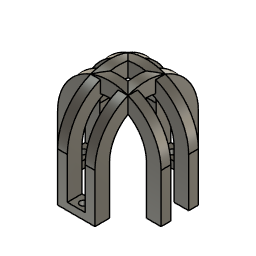
final motor guard (Autodesk Fusion 360 design; units mm, degrees)
Autodesk Fusion 360 part; units mm, degrees
note: some values were not read from the file. Chosen so that the rebuilt part matches the saved one: which bodies a step acts on.
sketch "Sketch1" plane through (0, 0, 0) normal (0, 0, 1) x (1, 0, 0) in component "guard"
  line L0 (-7.5594, 18.25) -> (-18.25, 7.5594)
  line L1 (-18.25, 7.5594) -> (-18.25, -7.5594)
  line L2 (-18.25, -7.5594) -> (-7.5594, -18.25)
  line L3 (-7.5594, -18.25) -> (7.5594, -18.25)
  line L4 (7.5594, -18.25) -> (18.25, -7.5594)
  line L5 (18.25, -7.5594) -> (18.25, 7.5594)
  line L6 (18.25, 7.5594) -> (7.5594, 18.25)
  line L7 (7.5594, 18.25) -> (-7.5594, 18.25)
  circle A0 centre (0, -18.25) radius 1.5
  line L8 (0, 0) -> (0, -18.25)
  circle A1 centre (18.25, 0) radius 1.5
  circle A2 centre (0, 18.25) radius 1.5
  circle A3 centre (-18.25, 0) radius 1.5
  line L9 (0, -18.25) -> (0, -21.25)
  line L10 (0, -21.25) -> (7.663, -21.25)
  line L11 (0, -21.25) -> (-7.663, -21.25)
  line L12 (21.25, 0) -> (21.25, -7.663)
  line L13 (21.25, 0) -> (21.25, 7.663)
  line L14 (18.25, 0) -> (21.25, 0)
  line L15 (0, 21.25) -> (7.663, 21.25)
  line L16 (0, 21.25) -> (-7.663, 21.25)
  line L17 (0, 18.25) -> (0, 21.25)
  line L18 (-21.25, 0) -> (-21.25, 7.663)
  line L19 (-21.25, 0) -> (-21.25, -7.663)
  line L20 (-18.25, 0) -> (-21.25, 0)
  line L21 (7.663, -21.25) -> (7.663, -15.25)
  line L22 (-7.663, -21.25) -> (-7.663, -15.25)
  line L23 (0, -18.25) -> (0, -15.25)
  line L24 (-7.663, -15.25) -> (-3.663, -15.25)
  line L25 (-3.663, -15.25) -> (-3.663, -21.25)
  line L26 (0, -18.25) -> (-3, -18.25)
  line L27 (7.663, -15.25) -> (3.663, -15.25)
  line L28 (3.663, -15.25) -> (3.663, -21.25)
  line L29 (-3.663, -15.25) -> (3.663, -15.25)
  line L30 (21.25, -7.663) -> (15.25, -7.663)
  line L31 (15.25, -7.663) -> (15.25, -3.663)
  line L32 (15.25, -3.663) -> (21.25, -3.663)
  line L33 (21.25, 0) -> (21.25, -7.663)
  line L34 (15.25, 7.663) -> (15.25, 3.663)
  line L35 (21.25, 7.663) -> (15.25, 7.663)
  line L36 (15.25, 3.663) -> (21.25, 3.663)
  line L37 (21.25, 0) -> (21.25, 7.663)
  line L38 (15.25, -3.663) -> (15.25, 3.663)
  line L39 (7.663, 21.25) -> (7.663, 15.25)
  line L40 (7.663, 15.25) -> (3.663, 15.25)
  line L41 (3.663, 15.25) -> (3.663, 21.25)
  line L42 (0, 21.25) -> (7.663, 21.25)
  line L43 (-7.663, 15.25) -> (-3.663, 15.25)
  line L44 (-7.663, 21.25) -> (-7.663, 15.25)
  line L45 (-3.663, 15.25) -> (-3.663, 21.25)
  line L46 (0, 21.25) -> (-7.663, 21.25)
  line L47 (3.663, 15.25) -> (-3.663, 15.25)
  line L48 (-21.25, 7.663) -> (-15.25, 7.663)
  line L49 (-15.25, 7.663) -> (-15.25, 3.663)
  line L50 (-15.25, 3.663) -> (-21.25, 3.663)
  line L51 (-21.25, 0) -> (-21.25, 7.663)
  line L52 (-15.25, -7.663) -> (-15.25, -3.663)
  line L53 (-21.25, -7.663) -> (-15.25, -7.663)
  line L54 (-15.25, -3.663) -> (-21.25, -3.663)
  line L55 (-21.25, 0) -> (-21.25, -7.663)
  line L56 (-15.25, 3.663) -> (-15.25, -3.663)
  dimension "d1" = 18.25
  dimension "d2" = 3
  dimension "d3" = 18.25
  dimension "d5" = 360
  dimension "d6" = 3
  dimension "d7" = 7.663
  dimension "d9" = 360
  dimension "d10" = 6
  dimension "d11" = 3
  dimension "d13" = 4
  dimension "d15" = 4
  dimension "d17" = 360
  constraint coincident L8.start origin
  constraint midpoint L3 A0.centre
  constraint coincident A0.centre L8.end
  constraint perpendicular L3 L9
  constraint vertical L9
  constraint perpendicular L9 L10
  constraint symmetric L10.start L9 L11.start
  constraint symmetric L9 L10.end L11.end
  constraint perpendicular L10 L21
  constraint symmetric L9 L21.end L22.end
  constraint perpendicular L3 L23
  constraint perpendicular L22 L24
  constraint coincident L11 L25.end
  constraint perpendicular L11 L25
  constraint perpendicular L9 L26
  constraint perpendicular L21 L27
  constraint coincident L10 L28.end
  constraint perpendicular L10 L28
  measures "d1" distance of L8.start L7
  measures "d2" diameter of A0
  measures "d3" vertical distance of L8.start A0.centre
  measures "d6" distance of A0.centre L9.end
  measures "d7" distance of L9.end L10.end
  measures "d10" distance of L10.end L21.end
  measures "d11" distance of A0.centre L23.end
  measures "d13" distance of L22.end L24.end
  measures "d15" distance of L21.end L27.end
extrude "Extrude1" add sketch "Sketch1" along normal blind 20 contours L0 L7 L43 L44 L45 | L0 L7 L16 L44 L45 L46 | L0 L1 L48 L49 L50 | L0 L1 L18 L48 L50 L51 | L6 L7 L39 L40 L41 | L6 L7 L15 L39 L41 L42 | L1 L2 L52 L53 L54 | L1 L2 L19 L53 L54 L55 | L5 L6 L13 L35 L36 L37 | L5 L6 L34 L35 L36 | L2 L3 L22 L24 L25 | L2 L3 L11 L22 L25 | L4 L5 L30 L31 L32 | L4 L5 L12 L30 L32 L33 | L3 L4 L10 L21 L28 | L3 L4 L21 L27 L28 makes body 1 at (-17.25, -3.663, 13.3333) makes body 2 at (3.663, 17.25, 13.3333) makes body 3 at (17.25, 3.663, 6.6667) makes body 4 at (-3.663, -17.25, 13.3333) makes body 5 at (-19.25, 7.663, 13.3333) makes body 6 at (-3.663, 17.25, 6.6667) makes body 7 at (17.25, -3.663, 6.6667) makes body 8 at (3.663, -17.25, 13.3333) in component "guard"
extrude "Extrude2" add sketch "Sketch1" along normal blind 3 contours L7 A2 L16 L17 L45 L46 | L7 A2 L41 L45 L47 | L7 A2 L15 L17 L41 L42 | L1 A3 L50 L54 L56 | L1 A3 L18 L20 L50 L51 | L1 A3 L19 L20 L54 L55 | L5 A1 L13 L14 L36 L37 | L5 A1 L32 L36 L38 | L5 A1 L12 L14 L32 L33 | L3 A0 L8 L23 L25 L26 L29 | L3 A0 L9 L11 L25 L26 | L3 A0 L9 L10 L28 | L3 A0 L8 L23 L28 L29 bodies 1 2 3 4 5 6 7 8 in component "guard"
extrude "Extrude3" cut 1 faces at (2.942, -18.25, 3) along direction (0, 0, -1) blind 18 on bodies 4 bodies 4 makes body 9 at (-3.663, -17.25, 13.3333) in component "guard"
sketch "Sketch2" plane through (0, -7.663, 0) normal (0, -1, 0) x (1, 0, 0) in component "guard"
  line L0 (-21.25, 0) -> (-15.25, 0)
  line L1 (-15.25, 0) -> (-15.25, 20)
  line L2 (-15.25, 20) -> (-21.25, 20)
  line L3 (-21.25, 20) -> (-21.25, 0)
  arc A0 (15.25, 20) -> (-15.25, 20) centre (0, 20) ccw
  arc A1 (21.25, 20) -> (-21.25, 20) centre (0, 20) ccw
  line L4 (15.25, 0) -> (15.25, 20)
  line L5 (21.25, 0) -> (21.25, 20)
  line L6 (-21.25, 20) -> (-15.25, 20)
  line L7 (15.25, 20) -> (21.25, 20)
  constraint coincident L1.end L2.start
  constraint tangent L1 A0
  constraint coincident L2.end L3.start
  constraint tangent L3 A1
  constraint coincident A0.start L4
  constraint coincident A1.start L5
  constraint coincident A1.start L5.end
  constraint perpendicular L5 L7
extrude "Extrude4" add sketch "Sketch2" along normal blind -15.326 and the other way blind 11.326 contours L2 A0 A1 L6 L7 bodies 1 3 in component "guard"
extrude "Extrude5" add sketch "Sketch2" against normal blind 4 contours L2 A0 A1 L6 L7 bodies 1 in component "guard"
sketch "Sketch3" plane through (7.663, 0, 0) normal (1, 0, 0) x (0, 1, 0) in component "guard"
  line L0 (-21.25, 0) -> (-15.25, 0)
  line L1 (-15.25, 0) -> (-15.25, 20)
  line L2 (-15.25, 20) -> (-21.25, 20)
  line L3 (-21.25, 20) -> (-21.25, 0)
  arc A0 (15.25, 20) -> (-15.25, 20) centre (0, 20) ccw
  arc A1 (21.25, 20) -> (-21.25, 20) centre (0, 20) ccw
  line L4 (-21.25, 20) -> (-15.25, 20)
  line L5 (15.25, 20) -> (21.25, 20)
  line L6 (21.25, 0) -> (21.25, 20)
  line L7 (15.25, 0) -> (15.25, 20)
  constraint coincident L1.end L2.start
  constraint tangent L1 A0
  constraint coincident L2.end L3.start
  constraint tangent L3 A1
  constraint parallel L4 L5
  constraint coincident A1.start L6
  constraint coincident A0.start L7
extrude "Extrude6" add sketch "Sketch3" against normal blind 4 contours L2 A0 A1 L4 L5 bodies 1 2 4 in component "guard"
extrude "Extrude7" add sketch "Sketch3" along normal blind -11.326 and the other way blind 15.326 contours L2 A0 A1 L4 L5 bodies 1 9 in component "guard"
extrude "Extrude8" add sketch "Sketch1" along normal blind 3 contours L3 A0 L8 L23 L25 L26 L29 | L3 A0 L9 L11 L25 L26 | L3 A0 L9 L10 L28 | L3 A0 L8 L23 L28 L29 bodies 1 in component "guard"
extrude "Extrude9" cut 1 faces at (18.2874, 2.9406, 3) along direction (0, 0, -1) blind 13 on bodies 1 bodies 1 in component "guard"
component "guard" placed x (1, 0, 0) y (0, 1, 0) z (0, 0, 1) at (0, 0, 0)
